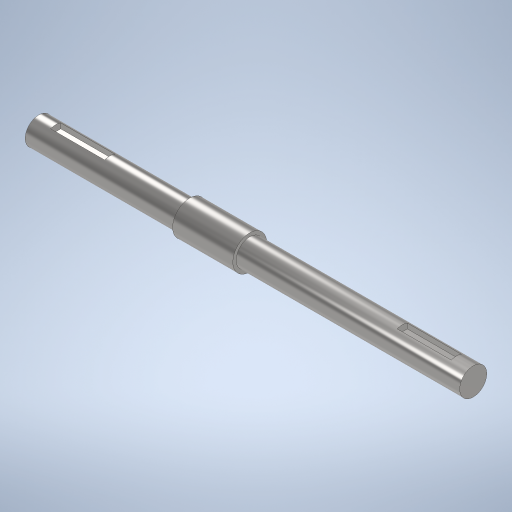
# Autodesk Inventor part: shoulder2_shaft
Saved by Autodesk Inventor 2024 (Build 280153000, 153)
## iProperties
Created: 2025-08-07
Part Number: shoulder2_shaft
Material: 鋼、炭素鋼
Document SubType Name: Modeling
Designer: HosodaLab2
Density: 7.85 g/cm^3
Appearance: 半つや出し
個数: 1
Author: HosodaLab2
Autodesk Inventor part; units mm, degrees
ref_plane "YZ Plane" through (0, 0, 0) normal (1, 0, 0) x (0, 1, 0)
ref_plane "XZ Plane" through (0, 0, 0) normal (0, 1, 0) x (-1, 0, 0)
ref_plane "XY Plane" through (0, 0, 0) normal (0, 0, 1) x (1, 0, 0)
sketch "スケッチ1" plane through (0, 0, 0) normal (0, 1, 0) x (-1, 0, 0)
  circle A0 centre (0, 0) radius 5
  dimension "d0" = 10
  constraints: 1 centre point, 1 coincident
  measures "d0" diameter of A0
extrude "押し出し1" add sketch "スケッチ1" along normal blind 17.8
sketch "スケッチ2" plane through (0, 17.8, 0) normal (0, 1, 0) x (1, 0, 0)
  circle A0 centre (0, 0) radius 4
  dimension "d3" = 8
  constraints: 1 centre point, 1 coincident
  measures "d3" diameter of A0
extrude "押し出し2" add sketch "スケッチ2" along normal blind 66.1
sketch "スケッチ3" plane through (0, 0, 0) normal (0, -1, 0) x (1, 0, 0)
  circle A0 centre (0, 0) radius 4
  dimension "d6" = 8
  constraints: 1 centre point, 1 coincident
  measures "d6" diameter of A0
extrude "押し出し3" add sketch "スケッチ3" along normal blind 44.6
sketch "スケッチ4" plane through (0, -44.6, 0) normal (0, -1, 0) x (1, 0, 0)
  circle A0 centre (0, 0) radius 4 projected
  point P0 (0, 4)
  constraints: 1 vertical alignment, 1 other
ref_plane "作業平面1" through (0, -44.6, 4) normal (0, 0, 1) x (1, 0, 0)
sketch "スケッチ7" plane through (0, -44.6, 4) normal (0, 0, 1) x (1, 0, 0)
  line L0 (-1.5, 5) -> (1.5, 5)
  line L1 (1.5, 5) -> (1.5, 21)
  line L2 (1.5, 21) -> (-1.5, 21)
  line L3 (-1.5, 21) -> (-1.5, 5)
  line L4 (-1.5, 5) -> (1.5, 21) construction
  line L5 (1.5, 5) -> (-1.5, 21) construction
  line L6 (-4, 0) -> (4, 0) projected
  line L7 (-1.5, 107.5) -> (1.5, 107.5)
  line L8 (1.5, 107.5) -> (1.5, 123.5)
  line L9 (1.5, 123.5) -> (-1.5, 123.5)
  line L10 (-1.5, 123.5) -> (-1.5, 107.5)
  line L11 (-1.5, 107.5) -> (1.5, 123.5) construction
  line L12 (1.5, 107.5) -> (-1.5, 123.5) construction
  line L13 (4, 128.5) -> (-4, 128.5) projected
  point P0 (0, 44.6)
  point P1 (0, 13)
  point P2 (0, 115.5)
  dimension "d17" = 3
  dimension "d18" = 16
  dimension "d19" = 5
  dimension "d20" = 3
  dimension "d21" = 16
  dimension "d22" = 5
  constraints: 24 end point, 4 midpoint, 4 parallel, 2 horizontal, 2 perpendicular
  measures "d17" distance of L2.end L1.end
  measures "d18" distance of L1.end L0.end
  measures "d19" distance between parallel lines of L6 L0
  measures "d20" distance of L9.end L8.end
  measures "d21" distance of L8.end L7.end
  measures "d22" distance between parallel lines of L13 L9
extrude "押し出し5" cut sketch "スケッチ7" against normal blind 1.8
